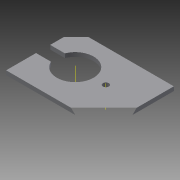
# Autodesk Inventor part: GehäuseFront
Saved by Autodesk Inventor 2014 (Build 180170000, 170)
## iProperties
Created: 2013-05-31
Part Number: GehäuseFront
Material: Generisch
Document SubType Name: Modeling
Designer: hanse
Density: 1 g/cm^3
Appearance: Vorgabe
Author: hanse
Autodesk Inventor part; units mm, degrees
ref_plane "YZ Plane" through (0, 0, 0) normal (1, 0, 0) x (0, 1, 0)
ref_plane "XZ Plane" through (0, 0, 0) normal (0, 1, 0) x (-1, 0, 0)
ref_plane "XY Plane" through (0, 0, 0) normal (0, 0, 1) x (1, 0, 0)
sketch "Skizze1" plane through (0, 0, 0) normal (0, 0, 1) x (1, 0, 0)
  line L0 (0, 0) -> (47.7997, 0)
  line L1 (47.7997, 0) -> (47.7997, 34.2455)
  line L2 (47.7997, 34.2455) -> (0, 34.2455)
  line L3 (0, 34.2455) -> (0, 0)
  circle A0 centre (15.5546, 18.2455) radius 1.05
  circle A1 centre (30.5546, 18.2455) radius 1.45
  line L4 (0, 18.2455) -> (47.7997, 18.2455)
  dimension "d0" = 2.1
  dimension "d1" = 2.9
  dimension "d2" = 15
  dimension "d16" = 16
  constraints: 10 end point, 4 point on line, 2 centre point, 2 parallel, 2 perpendicular, 1 horizontal
  measures "d0" diameter of A0
  measures "d1" diameter of A1
  measures "d2" distance of A1.centre A0.centre
  measures "d16" distance between parallel lines of L2 L4
extrude "Extrusion1" add sketch "Skizze1" along normal blind 2 contours L3 L4 A0 A1 L1 L0 | L3 L2 L1 L4 A1 A0
sketch "Skizze5" plane through (0, 0, 2) normal (0, 0, 1) x (1, 0, 0)
  circle A0 centre (15.5546, 18.2455) radius 1.05 projected
  circle A1 centre (15.5546, 18.2455) radius 9
  line L0 (10.0196, 14.6319) -> (-2.5086, 14.6319)
  line L1 (-2.5086, 14.6319) -> (-2.5086, 21.5511)
  line L2 (-2.5086, 21.5511) -> (10.0196, 21.5511)
  line L3 (10.0196, 21.5511) -> (10.0196, 14.6319)
  circle A2 centre (15.5546, 18.2455) radius 7.5 projected
  dimension "d24" = 1.5
  constraints: 8 end point, 2 parallel, 1 centre point, 1 coincident, 1 horizontal, 1 perpendicular
  measures "d24" radial gap between concentric circles of A1 A2
extrude "Extrusion5" cut sketch "Skizze5" against normal through all
